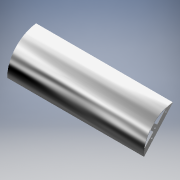
# Autodesk Inventor part: Kick Plate
Saved by Autodesk Inventor 2017 (Build 210142000, 142)
## iProperties
Created: 2017-01-14
Part Number: Kick Plate
Material: Generic
Document SubType Name: Modeling
Designer: Ben
Density: 1 g/cm^3
Appearance: Chrome - Polished
Author: Ben
Autodesk Inventor part; units mm, degrees
ref_plane "YZ Plane" through (0, 0, 0) normal (1, 0, 0) x (0, 1, 0)
ref_plane "XZ Plane" through (0, 0, 0) normal (0, 1, 0) x (-1, 0, 0)
ref_plane "XY Plane" through (0, 0, 0) normal (0, 0, 1) x (1, 0, 0)
sketch "Sketch1" plane through (0, 0, 0) normal (1, 0, 0) x (0, 1, 0)
  arc A0 (145.7933, 17.9012) -> (0, 146.8882) centre (0, 0) ccw
  line L0 (0, 0) -> (145.7933, 17.9012) construction
  line L1 (0, 0) -> (0, 146.8882) construction
  arc A1 (147.369, 18.0946) -> (0, 148.4757) centre (0, 0) ccw
  line L2 (0, 146.8882) -> (0, 148.4757)
  line L3 (145.7933, 17.9012) -> (147.369, 18.0946)
  dimension "d0" = 146.8882
  dimension "d1" = 83
  dimension "d2" = 1.5875
  constraints: 8 end point, 4 point on circle, 2 centre point, 2 vertical, 1 coincident, 1 collinear
  measures "d0" radius of A0
  measures "d1" angle of L1 L0
  measures "d2" radial gap between concentric circles of A0 A1
extrude "Extrusion1" add sketch "Sketch1" along normal blind 612.775
sketch "Sketch2" plane through (612.775, 0, 0) normal (1, 0, 0) x (0, 0, -1)
  arc A0 (-17.9012, 145.7933) -> (-146.8882, 0) centre (0, 0) ccw construction
  line L0 (-146.8882, 0) -> (0, 0) construction
  line L1 (-17.9012, 145.7933) -> (0, 0) construction
  line L2 (0, 0) -> (-110.0128, 97.3311) construction
  circle A1 centre (-97.8275, 86.5505) radius 3.175
  arc A2 (-18.0946, 147.369) -> (-148.4757, 0) centre (0, 0) ccw projected
  line L3 (-146.8882, 0) -> (-17.9012, 145.7933)
  line L4 (-48.0247, 140.4943) -> (-88.247, 95.0313)
  line L5 (-88.247, 95.0313) -> (-102.3789, 107.5341)
  line L6 (-105.0776, 76.0078) -> (-119.2095, 88.5107)
  line L7 (-89.4123, 96.0622) -> (-106.2428, 77.0388) construction
  line L8 (-88.247, 95.0313) -> (-105.0776, 76.0078) construction
  line L9 (-105.0776, 76.0078) -> (-145.2999, 30.5448)
  arc A3 (-102.3789, 107.5341) -> (-119.2095, 88.5107) centre (0, 0) ccw
  arc A4 (-145.2999, 30.5448) -> (-148.4757, 0) centre (0, 0) ccw
  line L10 (-148.4757, 0) -> (-146.8882, 0) projected
  line L11 (-146.8882, 0) -> (-148.4757, 0)
  arc A5 (-18.0946, 147.369) -> (-48.0247, 140.4943) centre (0, 0) ccw
  line L12 (-17.9012, 145.7933) -> (-18.0946, 147.369) projected
  line L13 (-18.0946, 147.369) -> (-17.9012, 145.7933)
  line L14 (-89.5285, 79.2081) -> (-112.9073, 52.7832) construction
  line L15 (-105.7735, 46.4717) -> (-120.0411, 59.0946) construction
  circle A6 centre (-112.9073, 52.7832) radius 3.175
  line L16 (-112.9073, 52.7832) -> (-97.8275, 86.5505) construction
  line L17 (-97.8275, 86.5505) -> (-64.0602, 71.4707) construction
  line L18 (-55.4274, 132.1271) -> (-41.1598, 119.5042) construction
  circle A7 centre (-48.2936, 125.8156) radius 3.175
  line L19 (37.2889, 78.6069) -> (-112.9073, 52.7832)
  line L20 (37.2889, 78.6069) -> (-64.0602, 71.4707)
  dimension "d5" = 6.35
  dimension "d6" = 130.6186
  dimension "d7" = 25.4
  dimension "d8" = 19.05
  dimension "d13" = 6.35
  dimension "d18" = 11.0808
  dimension "d19" = 62.23
  dimension "d20" = 152.4
  dimension "d21" = 101.6
  constraints: 38 end point, 12 perpendicular, 11 point on circle, 9 point on line, 6 centre point, 4 coincident, 3 midpoint, 3 parallel, 1 equal radius, 1 horizontal
  measures "d5" diameter of A1
  measures "d6" distance of L16.end point (0, 0)
  measures "d7" distance between parallel lines of L6 L5
  measures "d8" distance between parallel lines of L3 L4
  measures "d13" diameter of A6
  measures "d18" distance from line of L16.end L14
  measures "d19" distance from line of L2 A7.centre
  measures "d20" distance of L19.start L16.start
  measures "d21" distance of L19.start L17.end
extrude "Extrusion2" add sketch "Sketch2" along normal blind 1.5875 contours L12 L3 L10 A2 L9 L6 L5 L4
sketch "Sketch3" plane through (0, 0, 0) normal (-1, 0, 0) x (0, 0, 1)
  arc A0 (146.8882, 0) -> (143.1353, 32.9914) centre (0, 0) ccw projected
  line L0 (105.0776, 76.0078) -> (143.1353, 32.9914) projected
  line L1 (118.0161, 87.4549) -> (105.0776, 76.0078) projected
  arc A1 (118.0161, 87.4549) -> (101.1855, 106.4783) centre (0, 0) ccw projected
  line L2 (88.247, 95.0313) -> (101.1855, 106.4783) projected
  line L3 (50.1893, 138.0477) -> (88.247, 95.0313) projected
  arc A2 (50.1893, 138.0477) -> (17.9012, 145.7933) centre (0, 0) ccw projected
  line L4 (146.8882, 0) -> (17.9012, 145.7933) projected
  circle A3 centre (97.8275, 86.5505) radius 3.175 projected
  arc A4 (146.8882, 0) -> (17.9012, 145.7933) centre (0, 0) ccw projected
  line L5 (146.8882, 0) -> (148.4757, 0) projected
  arc A5 (148.4757, 0) -> (18.0946, 147.369) centre (0, 0) ccw projected
  line L6 (18.0946, 147.369) -> (17.9012, 145.7933) projected
extrude "Extrusion3" add sketch "Sketch3" along normal blind 1.5875 contours L4 A2 L3 L2 A1 L1 L0 A0 | A0 A4 A1 A2 L6 A5 L5
body "Solid1"
